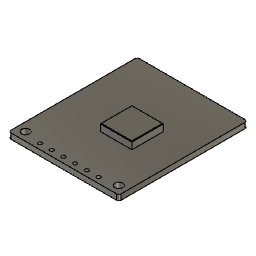
DFRobot SEN0395 Back Cover and Board Holder (Autodesk Fusion 360 archive; units mm, degrees)
design "DFRobot SEN0395"
Autodesk Fusion 360 part; units mm, degrees
sketch "Sketch1" plane through (0, 0, 0) normal (0, 0, 1) x (1, 0, 0)
  line L0 (0.5, 0) -> (23.5, 0)
  line L1 (24, 0.5) -> (24, 27.5)
  line L2 (23.5, 28) -> (0.5, 28)
  line L3 (0, 27.5) -> (0, 0.5)
  arc A0 (24, 27.5) -> (23.5, 28) centre (23.5, 27.5) ccw
  arc A1 (23.5, 0) -> (24, 0.5) centre (23.5, 0.5) ccw
  arc A2 (0, 0.5) -> (0.5, 0) centre (0.5, 0.5) ccw
  arc A3 (0.5, 28) -> (0, 27.5) centre (0.5, 27.5) ccw
  circle A4 centre (1.85, 1.85) radius 0.85
  circle A5 centre (22.15, 1.85) radius 0.85
  circle A6 centre (5.6247, 1.2368) radius 0.4068
  circle A7 centre (8.1747, 1.2368) radius 0.4068
  circle A8 centre (10.7247, 1.2368) radius 0.4068
  circle A9 centre (13.2747, 1.2368) radius 0.4068
  circle A10 centre (15.8247, 1.2368) radius 0.4068
  circle A11 centre (18.3747, 1.2368) radius 0.4068
  point P0 (24, 0)
  point P1 (0, 28)
  dimension "d1" = 24
  dimension "d2" = 28
  dimension "d3" = 0.5
  dimension "d4" = 0.85
  dimension "d5" = 0.85
  dimension "d14" = 12.75
  dimension "d15" = 0
  constraint horizontal L0
  constraint vertical L1
  constraint horizontal L2
  constraint vertical L3
  constraint tangent L1 A0
  constraint tangent L2 A0
  constraint coincident P0 L0
  constraint coincident P0 L1
  constraint tangent L0 A1
  constraint tangent L1 A1
  constraint equal A0 A1
  constraint coincident origin L0
  constraint coincident origin L3
  constraint tangent L0 A2
  constraint tangent L3 A2
  constraint equal A0 A2
  constraint coincident P1 L2
  constraint coincident P1 L3
  constraint tangent L2 A3
  constraint tangent L3 A3
  constraint equal A0 A3
  measures "d1" distance of origin P0
  measures "d2" distance of origin P1
  measures "d3" radius of A0
  measures "d4" radius of A4
  measures "d5" radius of A5
extrude "Extrude1" add sketch "Sketch1" along normal blind 1.1
ref_plane "WorkPlane1" through (12, 14, 1.1) normal (0, 0, 1) x (1, 0, 0)
sketch "Sketch2" plane through (12, 14, 1.1) normal (0, 0, 1) x (1, 0, 0)
  line L0 (-2, -14) -> (-2, -4) construction
  line L1 (-2, -4) -> (-12, -4) construction
  line L2 (-2, -4) -> (4.85, -4)
  line L3 (4.85, -4) -> (4.85, 2.85)
  line L4 (4.85, 2.85) -> (-2, 2.85)
  line L5 (-2, 2.85) -> (-2, -4)
  dimension "d19" = 10
  dimension "d20" = 10
  dimension "d21" = 6.85
  dimension "d22" = 6.85
  constraint vertical L0
  constraint perpendicular L0 L1
  constraint horizontal L2
  constraint vertical L3
  constraint horizontal L4
  constraint vertical L5
  measures "d19" distance of L0.end L1.end
  measures "d20" distance of L0.start L0.end
  measures "d21" distance of L0.end L2.end
  measures "d22" distance of L0.end L4.end
extrude "Extrude2" add sketch "Sketch2" along normal blind 1.55
fillet "Fillet1" radius 0.1 4 edges at (13.425, 10, 2.65) (10, 13.425, 2.65) (13.425, 16.85, 2.65) (16.85, 13.425, 2.65)
ref_plane "WorkPlane2" through (12, 14, 0) normal (0, 0, -1) x (-1, 0, 0)
sketch "Sketch3" plane through (12, 14, 0) normal (0, 0, -1) x (1, 0, 0)
  line L0 (0, 14) -> (0, 5)
  line L1 (-2.5199, 5.0116) -> (2.4801, 5.0116)
  line L2 (2.4801, 5.0116) -> (2.4801, -9.9884)
  line L3 (2.4801, -9.9884) -> (-2.5199, -9.9884)
  line L4 (-2.5199, -9.9884) -> (-2.5199, 5.0116)
  dimension "d28" = 9
  dimension "d29" = 5
  dimension "d30" = 15
  constraint vertical L0
  constraint horizontal L1
  constraint vertical L2
  constraint horizontal L3
  constraint vertical L4
  measures "d28" distance of L0.start L0.end
  measures "d29" distance of L1.start L1.end
  measures "d30" distance of L1.start L3.end
extrude "Extrude3" add sketch "Sketch3" along normal blind 1.1
move_face "OffsetFaces1" offset 0.1 1 faces at (20.2731, 13.0557, 0)
